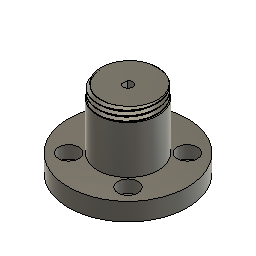
Base _part2 (Autodesk Fusion 360 design; units mm, degrees)
part number: 2025-04-16-17-35-49-953
Autodesk Fusion 360 part; units mm, degrees
sketch "Sketch1" plane through (0, 0, 0) normal (0, 1, 0) x (1, 0, 0)
  line L0 (20, 75) -> (-20, 75)
  line L1 (-100, 20) -> (-100, -20)
  line L2 (-20, -75) -> (20, -75)
  line L3 (100, -20) -> (100, 20)
  line L4 (20, 45.8258) -> (20, 75)
  line L5 (20, 75) -> (-20, 75)
  line L6 (-20, 75) -> (-20, 45.8258)
  line L7 (20, -45.8258) -> (20, -75)
  line L8 (20, -75) -> (-20, -75)
  line L9 (-20, -75) -> (-20, -45.8258)
  line L10 (45.8258, 20) -> (100, 20)
  line L11 (100, 20) -> (100, -20)
  line L12 (100, -20) -> (45.8258, -20)
  line L13 (-45.8258, 20) -> (-100, 20)
  line L14 (-100, 20) -> (-100, -20)
  arc A0 (45.8258, 20) -> (20, 45.8258) centre (0, 0) ccw
  arc A1 (-20, 45.8258) -> (-45.8258, 20) centre (0, 0) ccw
  line L15 (-100, -20) -> (-45.8258, -20)
  arc A2 (-45.8258, -20) -> (-20, -45.8258) centre (0, 0) ccw
  arc A3 (20, -45.8258) -> (45.8258, -20) centre (0, 0) ccw
  circle A4 centre (0, 0) radius 50
  dimension "d70" = 100
  constraint horizontal L0
  constraint perpendicular L0 L1
  constraint parallel L0 L2
  constraint parallel L1 L3
  constraint coincident A0.centre A1.centre
  constraint vertical L4
  constraint horizontal L5
  constraint vertical L6
  constraint vertical L7
  constraint horizontal L8
  constraint vertical L9
  constraint horizontal L10
  constraint vertical L11
  constraint horizontal L12
  constraint horizontal L13
  constraint vertical L14
  constraint horizontal L15
  constraint coincident L10.start A1
  constraint concentric A0 A1
  constraint concentric A1 A2
  constraint concentric A2 A3
  measures "d70" diameter of A1
extrude "Extrude1" add sketch "Sketch1" along normal blind 15 contours A0 A1 A2 A3 A4
sketch "Sketch3" plane through (0, 15, 0) normal (0, 1, 0) x (-1, 0, 0)
  circle A0 centre (0, 0) radius 50
  circle A1 centre (0, 0) radius 50
  dimension "d71" = 100
  constraint coincident A0.centre A1.centre
  measures "d71" diameter of A0
extrude "Extrude2" add sketch "Sketch3" along normal blind 10
sketch "Sketch5" plane through (0, 0, 0) normal (0, -1, 0) x (1, 0, 0)
  circle A0 centre (0, 0) radius 30
  circle A1 centre (0, 0) radius 50
  dimension "d72" = 60
  constraint coincident A0.centre A1.centre
  measures "d72" diameter of A0
extrude "Extrude4" cut sketch "Sketch5" against normal blind 10 contours A0
fillet "Fillet13" radius 5 1 edges at (-27.9698, 0, 10.8485)
sketch "Sketch6" plane through (0, 25, 0) normal (0, 1, 0) x (-1, 0, 0)
  circle A0 centre (0, 0) radius 50
  circle A1 centre (0, 0) radius 25.4
  circle A2 centre (0, 0) radius 10
  dimension "d44" = 20
  dimension "d49" = 50.8
  constraint coincident A0.centre A1.centre
  constraint concentric A1 A2
  measures "d44" diameter of A2
  measures "d49" diameter of A1
extrude "Extrude5" add sketch "Sketch6" along normal blind 40 contours A1
sketch "Sketch7" plane through (0, 65, 0) normal (0, 1, 0) x (-1, 0, 0)
  circle A0 centre (0, 0) radius 10
  circle A1 centre (0, 0) radius 25.4
  circle A2 centre (0, 0) radius 23
  constraint concentric A0 A2
extrude "Extrude6" add sketch "Sketch7" against normal blind 10 contours A0
extrude "Extrude7" add sketch "Sketch7" along normal blind 10 contours A0 | A2
thread "Thread2" "ISO Metric profile 50.0 M50x4 6g" major diameter 49.7025 minor diameter 45.1258 pitch 4 angle 60 modelled right hand crest width 0.569 on face at (-22.9714, 71.6667, -1.1465) crest through (-24.8513, 64, 0)
sketch "Sketch8" plane through (0, 0, 0) normal (0, 0, 1) x (1, 0, 0)
  line L0 (-105, 25) -> (-105, 145)
  dimension "d56" = 120
  constraint vertical L0
  measures "d56" distance of L0.start L0.end
sketch "Sketch9" plane through (0, 0, 0) normal (0, 1, 0) x (1, 0, 0)
  circle A0 centre (0, 175) radius 25
  line L0 (-17.3205, 205) -> (-34.641, 175)
  line L1 (-34.641, 175) -> (-17.3205, 145)
  line L2 (-17.3205, 145) -> (17.3205, 145)
  line L3 (17.3205, 145) -> (34.641, 175)
  line L4 (34.641, 175) -> (17.3205, 205)
  line L5 (17.3205, 205) -> (-17.3205, 205)
  point P0 (0, 175)
  dimension "d57" = 50
  constraint coincident P0 A0.centre
  measures "d57" diameter of A0
sketch "Sketch10" plane through (0, 75, 0) normal (0, 1, 0) x (-1, 0, 0)
  spline S0 degree 3 poles (-13.0991, 18.3711) (-15.5917, 16.7714) (-17.7447, 14.6962) (-21.1749, 9.7968) (-22.4016, 7.0081) (-23.7396, 1.0643) (-23.8173, -2.0377) (-22.7799, -8.1546) (-21.6541, -11.1066) (-18.8734, -15.5677) (-17.5164, -17.2162) (-14.3934, -20.1391) (-12.6364, -21.3961) (-10.7395, -22.4109) knots 0 0 0 0 0.88856 0.88856 1.793512 1.793512 2.71485 2.71485 3.652568 3.652568 4.289408 4.289408 4.933651 4.933651 4.933651 4.933651
  arc A0 (-10.7395, -22.4109) -> (10.7395, -22.4109) centre (0, 0) ccw
  spline S1 degree 3 poles (10.7395, -22.4109) (13.5662, -20.8988) (16.073, -18.8536) (20.1185, -13.9533) (21.6343, -11.1591) (23.4835, -5.1965) (23.819, -2.0921) (23.2758, 4.0148) (22.4233, 6.96) (20.1049, 11.4333) (18.9572, 13.0829) (16.2776, 16.0224) (14.7622, 17.3038) (13.0991, 18.3711) knots 0 0 0 0 0.961724 0.961724 1.907043 1.907043 2.83595 2.83595 3.748441 3.748441 4.349754 4.349754 4.943647 4.943647 4.943647 4.943647
  arc A1 (13.0991, 18.3711) -> (-13.0991, 18.3711) centre (0, 0) ccw
  line L0 (3, -2.6458) -> (3, 2.6458)
  arc A2 (3, 2.6458) -> (3, -2.6458) centre (0, 0) ccw
  dimension "d66" = 8
  constraint coincident A0.centre A1.centre
  measures "d66" diameter of A2
extrude "Extrude9" cut sketch "Sketch10" against normal blind 18 contours L0 A2
sketch "Sketch11" plane through (0, 0, 0) normal (0, 0, 1) x (1, 0, 0)
  line L0 (70, 0) -> (-70, 0)
  line L1 (-70, 0) -> (-70, 10)
  line L2 (-70, 10) -> (70, 10)
  line L3 (70, 10) -> (70, 0)
  dimension "d77" = 10
  constraint horizontal L0
  constraint vertical L1
  constraint horizontal L2
  constraint vertical L3
  measures "d77" distance of L0.start L2.end
extrude "Extrude10" cut sketch "Sketch11" along normal mid plane 170
sketch "Sketch12" plane through (0, 25, 0) normal (0, 1, 0) x (-1, 0, 0)
  circle A0 centre (0, 0) radius 50
  circle A1 centre (0, 0) radius 25.4
  line L0 (0, 0) -> (40, -40)
  line L1 (0, 0) -> (56.5685, 0) construction
  circle A2 centre (25, -25) radius 5
  circle A3 centre (25, -25) radius 8.5
  circle A4 centre (25, 25) radius 8.5
  circle A5 centre (25, 25) radius 5
  circle A6 centre (-25, 25) radius 8.5
  circle A7 centre (-25, 25) radius 5
  circle A8 centre (-25, -25) radius 8.5
  circle A9 centre (-25, -25) radius 5
  dimension "d80" = 45
  dimension "d81" = 10
  dimension "d82" = 25
  dimension "d83" = 17
  dimension "d85" = 360
  constraint horizontal L1
  constraint coincident A0.centre A1.centre
  constraint coincident L0 A2.centre
  constraint concentric A2 A3
  measures "d80" angle of L0 L1
  measures "d81" diameter of A2
  measures "d82" horizontal distance of A0.centre A2.centre
  measures "d83" diameter of A3
extrude "Extrude11" cut sketch "Sketch12" against normal blind 35 contours L0 A2 | L0 A2 | A5 | A7 | A9
extrude "Extrude12" cut sketch "Sketch12" against normal blind 10.5 contours L0 A2 A3 | L0 A2 A3 | A4 | A6 | A8
